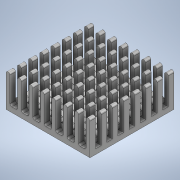
# Autodesk Inventor part: Heatsink_25x25x10
Saved by Autodesk Inventor 2020.1 (Build 241239000, 239)
## iProperties
Created: 2020-03-19
Part Number: Heatsink_25x25x10
Material: Generic
Document SubType Name: Modeling
Designer: yusaku
Density: 1 g/cm^3
Appearance: Anodized - Light Gray
Author: yusaku
Autodesk Inventor part; units mm, degrees
ref_plane "YZ Plane" through (0, 0, 0) normal (1, 0, 0) x (0, 1, 0)
ref_plane "XZ Plane" through (0, 0, 0) normal (0, 1, 0) x (-1, 0, 0)
ref_plane "XY Plane" through (0, 0, 0) normal (0, 0, 1) x (1, 0, 0)
sketch "Sketch1" plane through (0, 0, 0) normal (0, 0, 1) x (1, 0, 0)
  line L0 (0, 0) -> (12.5, 0)
  line L1 (12.5, 0) -> (12.5, 10)
  line L2 (12.5, 10) -> (11.3636, 10)
  line L3 (11.3636, 10) -> (11.3636, 1.5)
  line L4 (11.3636, 1.5) -> (9.0909, 1.5)
  line L5 (9.0909, 1.5) -> (9.0909, 10)
  line L6 (9.0909, 10) -> (7.9545, 10)
  line L7 (7.9545, 10) -> (7.9545, 1.5)
  line L8 (7.9545, 1.5) -> (5.6818, 1.5)
  line L9 (5.6818, 1.5) -> (5.6818, 10)
  line L10 (5.6818, 10) -> (4.5455, 10)
  line L11 (4.5455, 10) -> (4.5455, 1.5)
  line L12 (4.5455, 1.5) -> (2.2727, 1.5)
  line L13 (2.2727, 1.5) -> (2.2727, 10)
  line L14 (2.2727, 10) -> (1.1364, 10)
  line L15 (1.1364, 10) -> (1.1364, 1.5)
  line L16 (0, 1.5) -> (0, 0)
  line L17 (1.1364, 1.5) -> (-1.1364, 1.5)
  dimension "d0" = 12.5
  dimension "d1" = 10
  dimension "d2" = 1.1364
  dimension "d3" = 1.5
  constraints: 36 end point, 10 point on line, 9 perpendicular, 7 equal length, 3 vertical, 2 horizontal, 1 midpoint
  measures "d0" distance of L0.start L0.end
  measures "d1" distance of L0.end L1.end
  measures "d2" distance of L5.end L6.end
  measures "d3" distance of L16.start L0.start
extrude "Extrusion1" add sketch "Sketch1" along normal mid plane 25
fillet "Fillet1" radius 0.5682 15 edges at (11.3636, 10, 0) (11.3636, 1.5, 0) (9.0909, 1.5, 0) (9.0909, 10, 0) (7.9545, 10, 0) (7.9545, 1.5, 0) (5.6818, 1.5, 0) (5.6818, 10, 0) (4.5455, 10, 0) (4.5455, 1.5, 0) (2.2727, 1.5, 0) (2.2727, 10, 0) (1.1364, 10, 0) (1.1364, 1.5, 0) (12.5, 10, 0)
mirror "Mirror1" about plane through (0, 1.5, 0) normal (-1, 0, 0)
sketch "Sketch2" plane through (0, 0, 0) normal (1, 0, 0) x (0, 1, 0)
  line L0 (1.5, -12.5) -> (1.5, 12.5) projected
  line L1 (10, 10.8333) -> (1.5, 10.8333)
  line L2 (1.5, 10.8333) -> (1.5, 9.1667)
  line L3 (1.5, 9.1667) -> (10, 9.1667)
  line L4 (10, 9.1667) -> (10, 10.8333)
  line L5 (9.4318, 12.5) -> (2.0682, 12.5) projected
  line L6 (10, 10.8333) -> (10, 12.5)
  line L7 (0, -12.5) -> (0, 12.5) projected
  point P0 (0, 0)
  dimension "d7" = 3.3333
  dimension "d8" = 10
  constraints: 10 end point, 2 parallel, 2 point on line, 1 collinear, 1 horizontal, 1 perpendicular, 1 vertical
  measures "d7" distance between parallel lines of L5 L3
  measures "d8" distance between parallel lines of L7 L6
extrude "Extrusion2" cut sketch "Sketch2" along normal through all both and the other way through all
pattern_linear "Rectangular Pattern1" count 7 spacing 3.3333 along (0, 0, -1) of "Extrusion2"
body "Solid1"
